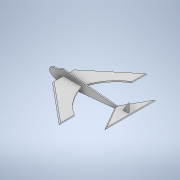
# Autodesk Inventor part: Airplane
Saved by Autodesk Inventor 2021 (Build 250183000, 183)
## iProperties
Created: 2020-07-09
Part Number: Airplane
Material: Generic
Document SubType Name: Modeling
Designer: saipr
Density: 1 g/cm^3
Appearance: Default
Author: saipr
Autodesk Inventor part; units mm, degrees
ref_plane "YZ Plane" through (0, 0, 0) normal (1, 0, 0) x (0, 1, 0)
ref_plane "XZ Plane" through (0, 0, 0) normal (0, 1, 0) x (-1, 0, 0)
ref_plane "XY Plane" through (0, 0, 0) normal (0, 0, 1) x (1, 0, 0)
sketch "Sketch6" plane through (0, 0, 0) normal (0, 0, 1) x (1, 0, 0)
  ellipse E0 centre (0, 0) end of major axis (38.1, 0) minor radius 19.05
  line L0 (-38.1, 0) -> (190.5, 0)
  line L1 (0, 19.05) -> (190.5, 0)
  line L2 (0, -19.05) -> (190.5, 0)
  line L3 (190.5, 0) -> (190.5, 28.9112)
  line L4 (190.5, 28.9112) -> (173.8081, 0)
  arc A0 (-26.467, 10.2187) -> (-38.1, 0) centre (-26.3616, -1.6322) ccw
  arc A1 (-26.467, 10.2187) -> (0, 19.05) centre (-26.8701, 55.5027) ccw
  point P0 (174.7192, 1.5781)
  dimension "d24" = 38.1
  dimension "d25" = 19.05
  dimension "d39" = 60
  constraints: 10 end point, 4 point on circle, 2 centre point, 1 coincident, 1 horizontal, 1 point on line, 1 tangent, 1 vertical, 5 other
  measures "d39" angle of L0 L4
sketch "Sketch7" plane through (0, 0, 0) normal (0, 1, 0) x (-1, 0, 0)
  line L0 (36.9474, -0.076) -> (-116.0592, 127.3834)
  line L1 (-116.0592, 127.3834) -> (-116.0592, -126.9058)
  line L2 (-116.0592, -126.9058) -> (36.9474, -0.076)
  line L3 (-194.7978, 0) -> (-194.7978, -74.0684)
  line L4 (-194.7978, -74.0684) -> (-152.0344, 0)
  line L5 (-152.0344, 0) -> (-194.7978, 74.0684)
  line L6 (-194.7978, 74.0684) -> (-194.7978, 0)
  line L7 (0, 0) -> (0, -30.7023)
  line L8 (0, -30.7023) -> (36.9474, -0.076)
  line L9 (0, 30.7023) -> (0, 0)
  arc A0 (-116.0592, -83.4665) -> (-55.5257, 0) centre (-187.7524, 32.2125) ccw
  arc A1 (-55.5257, 0) -> (-116.0592, 83.4665) centre (-187.7524, -32.2125) ccw
  line L10 (-55.5257, 0) -> (-55.3317, 0)
  line L11 (-55.3317, 0) -> (-55.7647, 0)
  line L12 (0, 0) -> (-101.3575, 0)
  dimension "d36" = 30
  dimension "d37" = 85.5268
  dimension "d38" = 85.5268
  dimension "d53" = 136.0938
  dimension "d54" = 136.0938
  dimension "d55" = 103.1066
  dimension "d56" = 103.1066
  constraints: 26 end point, 7 point on line, 4 collinear, 4 point on circle, 3 vertical, 2 centre point, 2 horizontal
  measures "d36" angle of L3 L4
  measures "d37" distance of L3.end L4.end
  measures "d38" distance of L4.end L5.end
  measures "d53" radius of A0
  measures "d54" radius of A1
  measures "d55" distance of L10.start A1.end
  measures "d56" distance of L10.start A0.start
extrude "Extrusion4" add sketch "Sketch7" along normal blind 3.175 contours L9 L12 L10 A1 L1 L0 | L2 L1 A0 L10 L12 L7 | L6 L5 L4 L3
extrude "Extrusion5" add sketch "Sketch6" along normal mid plane 3.175 contours L4 L3 L1
chamfer "Chamfer2" distance 3.175 angle 45 4 edges at (58.0296, 3.175, 79.0428) (58.0296, 3.175, -78.8041) (173.4161, 3.175, -37.0342) (173.4161, 3.175, 37.0342)
extrude "Extrusion6" cut sketch "Sketch7" along normal blind 76.2 contours L2 L7 L9 L0
extrude "Extrusion7" add sketch "Sketch6" along normal mid plane 3.175 contours L1 E0 L0 A0 A1 | L0 E0 L2 | L1 L4 L0 E0 | L0 L2 E0 | L1 L0 L4
chamfer "Chamfer3" distance 3.175 angle 45 2 edges at (0, 3.175, 14.0788) (0, 3.175, -14.083)
equation "\"d38\" = d37"
equation "\"d54\" = d53"
equation "\"d56\" = d55"
body "Solid3"
